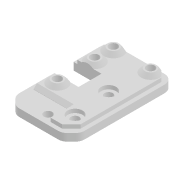
# Autodesk Inventor part: Print_Parts_S_rev2
Saved by Autodesk Inventor 2020 (Build 240168000, 168)
## iProperties
Created: 2020-11-09
Part Number: Print_Parts_S_rev2
Material: 一般
Document SubType Name: Modeling
Designer: kenta iguchi
Density: 1 g/cm^3
Appearance: 既定
Author: kenta iguchi
Autodesk Inventor part; units mm, degrees
ref_plane "YZ Plane" through (0, 0, 0) normal (1, 0, 0) x (0, 1, 0)
ref_plane "XZ Plane" through (0, 0, 0) normal (0, 1, 0) x (-1, 0, 0)
ref_plane "XY Plane" through (0, 0, 0) normal (0, 0, 1) x (1, 0, 0)
sketch "スケッチ43" plane through (0, 0, 0) normal (0, 1, 0) x (-1, 0, 0)
  line L0 (0, 0) -> (35, 0)
  line L1 (35, 0) -> (35, -40)
  line L2 (35, -40) -> (0, -40)
  line L3 (0, -40) -> (0, 0)
  line L4 (35, -23.85) -> (20, -23.85)
  line L5 (20, -23.85) -> (20, -36.15)
  line L6 (20, -36.15) -> (35, -36.15)
  line L7 (35, -36.15) -> (35, -23.85)
  line L8 (20, -36.15) -> (35, -36.15)
  line L9 (35, -36.15) -> (35, -40)
  line L10 (35, -40) -> (20, -40)
  line L11 (20, -40) -> (20, -36.15)
  point P0 (20, -30)
  point P1 (20, -40)
  dimension "d198" = 40
  dimension "d200" = 12.3
  dimension "d202" = 10
  dimension "d203" = 20
  dimension "d286" = 35
  constraints: 24 end point, 6 parallel, 3 horizontal, 3 perpendicular, 1 midpoint, 1 point on line
  measures "d198" distance of L0.end L1.end
  measures "d200" distance of L4.end L5.end
  measures "d202" distance from line of L2 point (20, -30)
  measures "d203" distance from line of point (20, -30) L3
  measures "d286" distance of L1.end L2.end
extrude "押し出し34" add sketch "スケッチ43" along normal blind 6 contours L0 L1 L4 L5 L11 L2 L3 | L11 L6 L1 L2
sketch "スケッチ44" plane through (0, 6, 0) normal (0, 1, 0) x (1, 0, 0)
  line L0 (-35, 0) -> (0, 0) projected
  line L1 (0, 0) -> (0, 40) projected
  line L2 (0, 40) -> (-35, 40) projected
  line L3 (-35, 40) -> (-35, 36.15) projected
  line L4 (-35, 36.15) -> (-20, 36.15) projected
  line L5 (-20, 36.15) -> (-20, 23.85) projected
  line L6 (-20, 23.85) -> (-35, 23.85) projected
  line L7 (-35, 23.85) -> (-35, 0) projected
  point P0 (-14, 30)
  point P1 (-10, 30)
  dimension "d206" = 30
  dimension "d207" = 10
  dimension "d209" = 6
  constraints: 1 horizontal alignment
  measures "d206" distance from line of L0 point (-10, 30)
  measures "d207" distance from line of point (-10, 30) L1
  measures "d209" distance from line of L5 point (-14, 30)
hole "穴7" at (-10, 6, -30) direction (0, -1, 0) diameter 4.4 end through all counterbore diameter 8 counterbore depth 2
sketch "スケッチ45" plane through (0, 6, 0) normal (0, 1, 0) x (1, 0, 0)
  circle A0 centre (-10, 30) radius 4 projected
  line L0 (-20, 36.15) -> (-20, 23.85) projected
  line L1 (-20, 23.85) -> (-35, 23.85) projected
  line L2 (-35, 23.85) -> (-35, 0) projected
  line L3 (-35, 0) -> (0, 0) projected
  line L4 (0, 0) -> (0, 40) projected
  line L5 (0, 40) -> (-35, 40) projected
  line L6 (-35, 40) -> (-35, 36.15) projected
  line L7 (-35, 36.15) -> (-20, 36.15) projected
  line L8 (0, 0) -> (0, 40) projected
  line L9 (0, 40) -> (-35, 40)
  line L10 (-35, 40) -> (-35, 55)
  line L11 (-35, 55) -> (0, 55)
  line L12 (0, 55) -> (0, 40)
  point P0 (-35, 40)
  dimension "d217" = 15
  constraints: 8 end point, 2 parallel, 1 horizontal, 1 perpendicular, 1 vertical alignment
  measures "d217" distance of L9.end L10.end
extrude "押し出し35" add sketch "スケッチ45" against normal up to surface (6 mm away) contours L10 L11 L12 L5
sketch "スケッチ46" plane through (0, 6, 0) normal (0, 1, 0) x (1, 0, 0)
  circle A0 centre (-10, 30) radius 4 projected
  line L0 (-20, 36.15) -> (-20, 23.85) projected
  line L1 (-20, 23.85) -> (-35, 23.85) projected
  line L2 (-35, 23.85) -> (-35, 0) projected
  line L3 (-35, 0) -> (0, 0) projected
  line L4 (0, 0) -> (0, 55) projected
  line L5 (0, 55) -> (-35, 55) projected
  line L6 (-35, 55) -> (-35, 36.15) projected
  line L7 (-35, 36.15) -> (-20, 36.15) projected
  point P0 (-27.5, 20)
  point P1 (-27.5, 40)
  point P2 (-27.5, 50)
  point P3 (-7.5, 50)
  dimension "d220" = 20
  dimension "d223" = 20
  dimension "d224" = 10
  dimension "d232" = 10
  dimension "d233" = 7.5
  constraints: 2 vertical alignment, 1 horizontal alignment
  measures "d220" distance of point (-27.5, 40) point (-27.5, 20)
  measures "d223" distance of point (-27.5, 50) point (-7.5, 50)
  measures "d224" distance of point (-27.5, 50) point (-27.5, 40)
  measures "d232" vertical distance of A0.centre point (-27.5, 20)
  measures "d233" distance from line of point (-27.5, 50) L6
hole "穴8" at (-27.5, 6, -20) at (-27.5, 6, -40) at (-27.5, 6, -50) at (-7.5, 6, -50) direction (0, -1, 0) diameter 4.4 end through all
sketch "スケッチ47" plane through (0, 6, 0) normal (0, 1, 0) x (1, 0, 0)
  circle A0 centre (-27.5, 50) radius 2.2 projected
  circle A1 centre (-27.5, 20) radius 2.2 projected
  circle A2 centre (-27.5, 40) radius 2.2 projected
  circle A3 centre (-7.5, 50) radius 2.2 projected
  circle A4 centre (-10, 30) radius 4 projected
  line L0 (0, 0) -> (0, 55) projected
  line L1 (0, 55) -> (-35, 55) projected
  line L2 (-35, 55) -> (-35, 36.15) projected
  line L3 (-35, 36.15) -> (-20, 36.15) projected
  line L4 (-20, 36.15) -> (-20, 23.85) projected
  line L5 (-20, 23.85) -> (-35, 23.85) projected
  line L6 (-35, 23.85) -> (-35, 0) projected
  line L7 (-35, 0) -> (0, 0) projected
  point P0 (-27, 10)
  point P1 (-8, 10)
  dimension "d234" = 10
  dimension "d235" = 8
  dimension "d236" = 8
  constraints: 1 horizontal alignment
  measures "d234" distance from line of point (-8, 10) L7
  measures "d235" distance from line of point (-27, 10) L6
  measures "d236" distance from line of point (-8, 10) L0
hole "穴9" at (-8, 6, -10) direction (0, -1, 0) diameter 4.4 end through all counterbore diameter 8 counterbore depth 2
sketch "スケッチ48" plane through (0, 6, 0) normal (0, 1, 0) x (1, 0, 0)
  circle A0 centre (-8, 10) radius 4 projected
  circle A1 centre (-27.5, 50) radius 2.2 projected
  circle A2 centre (-27.5, 20) radius 2.2 projected
  circle A3 centre (-27.5, 40) radius 2.2 projected
  circle A4 centre (-7.5, 50) radius 2.2 projected
  circle A5 centre (-10, 30) radius 4 projected
  line L0 (0, 0) -> (0, 55) projected
  line L1 (0, 55) -> (-35, 55) projected
  line L2 (-35, 55) -> (-35, 36.15) projected
  line L3 (-35, 36.15) -> (-20, 36.15) projected
  line L4 (-20, 36.15) -> (-20, 23.85) projected
  line L5 (-20, 23.85) -> (-35, 23.85) projected
  line L6 (-35, 23.85) -> (-35, 0) projected
  line L7 (-35, 0) -> (0, 0) projected
  circle A6 centre (-7.5, 50) radius 3
  circle A7 centre (-27.5, 50) radius 2.2 projected
  circle A8 centre (-27.5, 50) radius 3
  circle A9 centre (-27.5, 40) radius 2.2 projected
  circle A10 centre (-27.5, 40) radius 3
  circle A11 centre (-27.5, 20) radius 2.2 projected
  circle A12 centre (-27.5, 20) radius 3
  dimension "d244" = 6
  dimension "d245" = 6
  dimension "d246" = 6
  dimension "d247" = 6
  constraints: 4 centre point, 4 coincident
  measures "d244" diameter of A6
  measures "d245" diameter of A8
  measures "d246" diameter of A10
  measures "d247" diameter of A12
extrude "押し出し36" add sketch "スケッチ48" along normal blind 2 contours A6 | A8 | A10 | A12
chamfer "面取り13" distance 2 angle 45 4 edges at (-30.5, 6, -50) (-30.5, 6, -40) (-10.5, 6, -50) (-30.5, 6, -20)
sketch "スケッチ49" plane through (0, 6, 0) normal (0, 1, 0) x (1, 0, 0)
  arc A0 (-30.6902, 23.85) -> (-24.3098, 23.85) centre (-27.5, 20) ccw projected
  line L0 (-30.6902, 23.85) -> (-35, 23.85) projected
  line L1 (-35, 23.85) -> (-35, 0) projected
  line L2 (-35, 0) -> (0, 0) projected
  line L3 (0, 0) -> (0, 55) projected
  line L4 (0, 55) -> (-7.5, 55) projected
  circle A1 centre (-7.5, 50) radius 5 projected
  line L5 (-7.5, 55) -> (-27.5, 55) projected
  arc A2 (-27.5, 45) -> (-27.5, 55) centre (-27.5, 50) ccw projected
  arc A3 (-24.3098, 36.15) -> (-27.5, 45) centre (-27.5, 40) ccw projected
  line L6 (-20, 36.15) -> (-20, 23.85) projected
  circle A4 centre (-8, 10) radius 4 projected
  circle A5 centre (-10, 30) radius 4 projected
  line L7 (0, 55) -> (-7.5, 55) projected
  line L8 (-35, 0) -> (0, 0) projected
  line L9 (0, 55) -> (-35, 55)
  line L10 (-35, 55) -> (-35, 0)
  line L11 (-35, 0) -> (0, 0)
  line L12 (0, 0) -> (0, 55)
  line L13 (-33, 2) -> (-33, 53)
  line L14 (-33, 53) -> (-2, 53)
  line L15 (-2, 53) -> (-2, 2)
  line L16 (-2, 2) -> (-33, 2)
  circle A6 centre (-27.5, 50) radius 3 projected
  arc A7 (-27.5, 55) -> (-27.5, 45) centre (-27.5, 50) ccw projected
  arc A8 (-27.5, 45) -> (-27.5, 55) centre (-27.5, 50) ccw projected
  line L17 (-24.3098, 36.15) -> (-20, 36.15) projected
  line L18 (-20, 23.85) -> (-24.3098, 23.85) projected
  point P0 (-31.5, 53)
  point P1 (-23.5, 53)
  point P2 (-11.5, 53)
  point P3 (-3.5, 53)
  dimension "d253" = 2
  constraints: 16 end point, 4 parallel, 2 perpendicular, 1 horizontal, 4 other
  measures "d253" distance between parallel lines of L10 L13
extrude "押し出し37" cut sketch "スケッチ49" along normal blind 2 contours A7 A2 L14 | A1 L14 picked at (-25.0988, 53.2796) picked at (-8.5679, 53.2796)
sketch "スケッチ50" plane through (0, 6, 0) normal (0, 1, 0) x (1, 0, 0)
  circle A0 centre (-10, 30) radius 4 projected
  circle A1 centre (-8, 10) radius 4 projected
  line L0 (-11.5, 53) -> (-3.5, 53) projected
  arc A2 (-11.5, 53) -> (-3.5, 53) centre (-7.5, 50) ccw projected
  arc A3 (-27.5, 45) -> (-30.6902, 36.15) centre (-27.5, 40) ccw projected
  arc A4 (-31.5, 53) -> (-27.5, 45) centre (-27.5, 50) ccw projected
  line L1 (-31.5, 53) -> (-23.5, 53) projected
  arc A5 (-27.5, 45) -> (-23.5, 53) centre (-27.5, 50) ccw projected
  arc A6 (-24.3098, 36.15) -> (-27.5, 45) centre (-27.5, 40) ccw projected
  line L2 (-20, 36.15) -> (-20, 23.85) projected
  arc A7 (-30.6902, 23.85) -> (-24.3098, 23.85) centre (-27.5, 20) ccw projected
  line L3 (-30.6902, 23.85) -> (-35, 23.85) projected
  line L4 (-35, 23.85) -> (-35, 0) projected
  line L5 (-35, 0) -> (0, 0) projected
  line L6 (0, 0) -> (0, 55) projected
  line L7 (0, 55) -> (-35, 55) projected
  line L8 (-35, 55) -> (-35, 36.15) projected
  line L9 (-35, 36.15) -> (-30.6902, 36.15) projected
  line L10 (-35, 55) -> (0, 55) projected
  line L11 (-35, 23.85) -> (-35, 0) projected
  line L12 (0, 55) -> (-35, 55)
  line L13 (-35, 55) -> (-35, 0)
  line L14 (-35, 0) -> (0, 0)
  line L15 (0, 0) -> (0, 55)
  line L16 (-33, 2) -> (-33, 53)
  line L17 (-33, 53) -> (-2, 53)
  line L18 (-2, 53) -> (-2, 2)
  line L19 (-2, 2) -> (-33, 2)
  line L20 (-24.3098, 36.15) -> (-20, 36.15) projected
  line L21 (-20, 23.85) -> (-24.3098, 23.85) projected
  point P0 (-33, 23.85)
  point P1 (-33, 36.15)
  point P2 (-3.5, 53)
  dimension "d256" = 2
  constraints: 16 end point, 4 parallel, 2 perpendicular, 1 horizontal, 3 other
  measures "d256" distance between parallel lines of L13 L16
extrude "押し出し38" cut sketch "スケッチ50" against normal blind 2 contours L17 L1 L16 L9 L8 L7 L6 L5 L4 L3 L19 L18 L0
chamfer "面取り14" distance 5 angle 45 4 edges at (-35, 2, 0) (-33, 5, -2) (0, 2, 0) (-2, 5, -2)
sketch "スケッチ51" plane through (0, 6, 0) normal (0, 1, 0) x (1, 0, 0)
  line L0 (-2, 7) -> (-7, 2) projected
  line L1 (-2, 7) -> (-2, 53) projected
  line L2 (-2, 53) -> (-3.5, 53) projected
  arc A0 (-11.5, 53) -> (-3.5, 53) centre (-7.5, 50) ccw projected
  arc A1 (-27.5, 45) -> (-23.5, 53) centre (-27.5, 50) ccw projected
  arc A2 (-24.3098, 36.15) -> (-27.5, 45) centre (-27.5, 40) ccw projected
  line L3 (-20, 36.15) -> (-20, 23.85) projected
  arc A3 (-30.6902, 23.85) -> (-24.3098, 23.85) centre (-27.5, 20) ccw projected
  line L4 (-30.6902, 23.85) -> (-33, 23.85) projected
  line L5 (-33, 23.85) -> (-33, 7) projected
  line L6 (-28, 2) -> (-33, 7) projected
  line L7 (-28, 2) -> (-7, 2) projected
  circle A4 centre (-10, 30) radius 4 projected
  circle A5 centre (-8, 10) radius 4 projected
  circle A6 centre (-17.5, 5) radius 2.2
  line L8 (-5, 0) -> (-30, 0) projected
  line L9 (-35, 36.15) -> (-35, 55) projected
  line L10 (-11.5, 53) -> (-23.5, 53) projected
  line L11 (-24.3098, 36.15) -> (-20, 36.15) projected
  line L12 (-20, 23.85) -> (-24.3098, 23.85) projected
  point P0 (0, 0)
  dimension "d262" = 4.4
  dimension "d263" = 5
  dimension "d264" = 17.5
  constraints: 1 centre point
  measures "d262" diameter of A6
  measures "d263" distance from line of A6.centre L8
  measures "d264" distance from line of A6.centre L9
extrude "押し出し39" cut sketch "スケッチ51" against normal blind 6 contours A6
sketch "スケッチ52" plane through (0, 6, 0) normal (0, 1, 0) x (1, 0, 0)
  circle A0 centre (-17.5, 5) radius 2.2 projected
  line L0 (-2, 7) -> (-7, 2) projected
  line L1 (-2, 7) -> (-2, 53) projected
  line L2 (-2, 53) -> (-3.5, 53) projected
  arc A1 (-11.5, 53) -> (-3.5, 53) centre (-7.5, 50) ccw projected
  line L3 (-11.5, 53) -> (-23.5, 53) projected
  arc A2 (-27.5, 45) -> (-23.5, 53) centre (-27.5, 50) ccw projected
  arc A3 (-24.3098, 36.15) -> (-27.5, 45) centre (-27.5, 40) ccw projected
  line L4 (-20, 36.15) -> (-20, 23.85) projected
  arc A4 (-30.6902, 23.85) -> (-24.3098, 23.85) centre (-27.5, 20) ccw projected
  line L5 (-30.6902, 23.85) -> (-33, 23.85) projected
  line L6 (-33, 23.85) -> (-33, 7) projected
  line L7 (-28, 2) -> (-33, 7) projected
  line L8 (-28, 2) -> (-7, 2) projected
  circle A5 centre (-10, 30) radius 4 projected
  circle A6 centre (-8, 10) radius 4 projected
  circle A7 centre (-17.5, 5) radius 2.2 projected
  circle A8 centre (-17.5, 5) radius 4.25
  line L9 (-21.75, 5) -> (-13.25, 5)
  line L10 (-13.25, 5) -> (-13.25, -3.911)
  line L11 (-13.25, -3.911) -> (-21.75, -3.911)
  line L12 (-21.75, -3.911) -> (-21.75, 5)
  line L13 (-24.3098, 36.15) -> (-20, 36.15) projected
  line L14 (-20, 23.85) -> (-24.3098, 23.85) projected
  point P0 (0, 0)
  point P1 (-21.75, 2)
  point P2 (-13.25, 2)
  dimension "d267" = 8.5
  constraints: 8 end point, 2 parallel, 2 point on circle, 1 centre point, 1 coincident, 1 horizontal, 1 perpendicular
  measures "d267" diameter of A8
extrude "押し出し40" cut sketch "スケッチ52" against normal up to surface (2 mm away) contours L9 A8 L8 A0 | A0 L9 A8 | L10 L8 A8 | A8 L8 L12
sketch "スケッチ54" plane through (0, 6, 0) normal (0, 1, 0) x (1, 0, 0)
  line L0 (-36.1734, 0) -> (-13.25, 0)
  line L1 (-13.25, 0) -> (-13.25, 12.5)
  line L2 (-13.25, 12.5) -> (-36.1734, 12.5)
  line L3 (-36.1734, 12.5) -> (-36.1734, 0)
  line L4 (-5, 0) -> (-30, 0) projected
  line L5 (-13.25, 5) -> (-13.25, 2) projected
  line L6 (-13.25, 2) -> (-7, 2) projected
  line L7 (-2, 7) -> (-7, 2) projected
  line L8 (-2, 7) -> (-2, 53) projected
  line L9 (-2, 53) -> (-3.5, 53) projected
  arc A0 (-11.5, 53) -> (-3.5, 53) centre (-7.5, 50) ccw projected
  line L10 (-11.5, 53) -> (-23.5, 53) projected
  arc A1 (-27.5, 45) -> (-23.5, 53) centre (-27.5, 50) ccw projected
  arc A2 (-24.3098, 36.15) -> (-27.5, 45) centre (-27.5, 40) ccw projected
  line L11 (-20, 36.15) -> (-20, 23.85) projected
  arc A3 (-30.6902, 23.85) -> (-24.3098, 23.85) centre (-27.5, 20) ccw projected
  line L12 (-30.6902, 23.85) -> (-33, 23.85) projected
  line L13 (-33, 23.85) -> (-33, 7) projected
  line L14 (-28, 2) -> (-33, 7) projected
  line L15 (-28, 2) -> (-21.75, 2) projected
  line L16 (-21.75, 2) -> (-21.75, 5) projected
  arc A4 (-13.25, 5) -> (-21.75, 5) centre (-17.5, 5) ccw projected
  circle A5 centre (-10, 30) radius 4 projected
  circle A6 centre (-8, 10) radius 4 projected
  line L17 (-24.3098, 36.15) -> (-20, 36.15) projected
  line L18 (-20, 23.85) -> (-24.3098, 23.85) projected
  point P0 (0, 0)
  point P1 (-33, 12.5)
  dimension "d273" = 12.5
  constraints: 8 end point, 2 parallel, 1 horizontal, 1 perpendicular, 1 vertical alignment
  measures "d273" distance between parallel lines of L4 L2
extrude "押し出し42" cut sketch "スケッチ54" against normal up to surface (2 mm away) contours L2 L1 A4 L16 L15 L14 L13
chamfer "面取り15" distance 2 angle 45 1 edges at (-23.125, 6, -12.5)
sketch "スケッチ57" plane through (0, 4, 0) normal (0, 1, 0) x (1, 0, 0)
  circle A0 centre (-17.5, 5) radius 2.2 projected
  line L0 (-35, 55) -> (0, 55) projected
  line L1 (0, 55) -> (0, 5) projected
  line L2 (0, 5) -> (-5, 0) projected
  line L3 (-5, 0) -> (-30, 0) projected
  line L4 (-30, 0) -> (-35, 5) projected
  line L5 (-35, 5) -> (-35, 23.85) projected
  line L6 (-35, 23.85) -> (-33, 23.85) projected
  line L7 (-33, 23.85) -> (-20, 23.85) projected
  line L8 (-20, 23.85) -> (-20, 36.15) projected
  line L9 (-20, 36.15) -> (-33, 36.15) projected
  line L10 (-33, 36.15) -> (-35, 36.15) projected
  line L11 (-35, 36.15) -> (-35, 55) projected
  line L12 (-33, 12.5) -> (-33, 23.85) projected
  line L13 (-13.25, 12.5) -> (-33, 12.5) projected
  line L14 (-13.25, 2) -> (-13.25, 12.5) projected
  line L15 (-7, 2) -> (-13.25, 2) projected
  line L16 (-2, 7) -> (-7, 2) projected
  line L17 (-2, 53) -> (-2, 7) projected
  line L18 (-33, 53) -> (-2, 53) projected
  line L19 (-33, 36.15) -> (-33, 53) projected
  circle A1 centre (-8, 10) radius 4 projected
  circle A2 centre (-8, 10) radius 2.2 projected
  circle A3 centre (-27.5, 50) radius 2.2 projected
  circle A4 centre (-27.5, 20) radius 2.2 projected
  circle A5 centre (-27.5, 40) radius 2.2 projected
  circle A6 centre (-7.5, 50) radius 2.2 projected
  circle A7 centre (-10, 30) radius 4 projected
  circle A8 centre (-10, 30) radius 2.2 projected
  line L20 (-32.9, 23.85) -> (-32.9, 12.6)
  line L21 (-32.9, 12.6) -> (-13.15, 12.6)
  line L22 (-13.15, 12.6) -> (-13.15, 2.1)
  line L23 (-13.15, 2.1) -> (-7.0414, 2.1)
  line L24 (-7.0414, 2.1) -> (-2.1, 7.0414)
  line L25 (-2.1, 7.0414) -> (-2.1, 52.9)
  line L26 (-2.1, 52.9) -> (-32.9, 52.9)
  line L27 (-32.9, 52.9) -> (-32.9, 36.15)
  point P0 (0, 0)
  dimension "d279" = 0.1
  constraints: 16 end point, 7 other
  measures "d279" distance between parallel lines of L18 L26
extrude "押し出し43" cut sketch "スケッチ57" along normal blind 6 contours L19 L18 L17 L16 L15 L14 L13 L12 L7 L20 L21 L22 L23 L24 L25 L26 L27 L9
chamfer "面取り16" distance 2.5 angle 45 4 edges at (-32.9, 5, -52.9) (-35, 2, -55) (0, 2, -55) (-2.1, 5, -52.9)
fillet "フィレット3" radius 5 8 edges at (0, 2, -52.5) (-2.5, 2, -55) (-32.5, 2, -55) (-35, 2, -52.5) (0, 2, -5) (-5, 2, 0) (-30, 2, 0) (-35, 2, -5)
